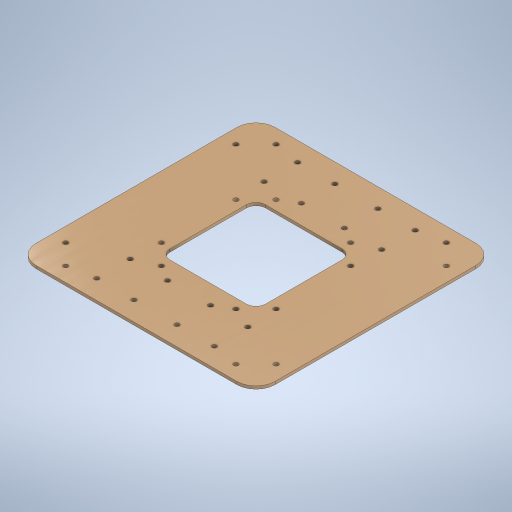
# Autodesk Inventor part: L1 Wood Base Iteration 1
Saved by Autodesk Inventor 2024 (Build 280153000, 153)
## iProperties
Created: 2023-06-26
Part Number: L1 Wood Base Iteration 1
Material: Aluminum 6061
Document SubType Name: Modeling
Designer: AdminForWorker
Density: 2.7 g/cm^3
Appearance: Brindle
Title: base
Author: AdminForWorker
Autodesk Inventor part; units mm, degrees
ref_plane "YZ Plane" through (0, 0, 0) normal (1, 0, 0) x (0, 1, 0)
ref_plane "XZ Plane" through (0, 0, 0) normal (0, 1, 0) x (-1, 0, 0)
ref_plane "XY Plane" through (0, 0, 0) normal (0, 0, 1) x (1, 0, 0)
sketch "Sketch3" plane through (0, 0, 0) normal (0, 1, 0) x (-1, 0, 0)
  line L0 (105, -125) -> (-105, -125)
  line L1 (-125, -105) -> (-125, 105)
  line L2 (-105, 125) -> (105, 125)
  line L3 (125, 105) -> (125, -105)
  line L4 (125, -125) -> (-125, 125) construction
  line L5 (-125, -125) -> (125, 125) construction
  arc A0 (125, 105) -> (105, 125) centre (105, 105) ccw
  arc A1 (105, -125) -> (125, -105) centre (105, -105) ccw
  arc A2 (-105, 125) -> (-125, 105) centre (-105, 105) ccw
  arc A3 (-125, -105) -> (-105, -125) centre (-105, -105) ccw
  line L6 (-40, 50) -> (40, 50)
  line L7 (50, 40) -> (50, -40)
  line L8 (40, -50) -> (-40, -50)
  line L9 (-50, -40) -> (-50, 40)
  line L10 (-50, 50) -> (50, -50) construction
  line L11 (50, 50) -> (-50, -50) construction
  arc A4 (50, 40) -> (40, 50) centre (40, 40) ccw
  arc A5 (-40, 50) -> (-50, 40) centre (-40, 40) ccw
  arc A6 (-50, -40) -> (-40, -50) centre (-40, -40) ccw
  arc A7 (40, -50) -> (50, -40) centre (40, -40) ccw
  point P0 (0, 0)
  dimension "L0" = 250
  dimension "W0" = 250
  dimension "d126" = 20
  dimension "d127" = 100
  dimension "d128" = 100
  dimension "d129" = 10
  constraints: 24 end point, 16 point on circle, 16 point on line, 16 tangent, 8 centre point, 6 equal radius, 4 midpoint, 4 parallel, 2 horizontal, 2 perpendicular
  measures "L0" distance of L4.end L5.end
  measures "W0" distance of L5.start L4.end
  measures "d126" radius of A0
  measures "d127" distance of L10.end L11.end
  measures "d128" distance of L11.start L10.end
  measures "d129" radius of A4
extrude "Main Body Extrusion" add sketch "Sketch3" along normal blind 3
sketch "Sketch11" plane through (0, 3, 0) normal (0, 1, 0) x (1, 0, 0)
  circle A0 centre (61.4917, -70.0531) radius 2.5
  circle A1 centre (22.4917, -105.0531) radius 2.5
  circle A2 centre (-22.5083, -70.0531) radius 2.5
  circle A3 centre (-61.5083, -105.0531) radius 2.5
  circle A4 centre (-22.5083, -105.0531) radius 2.5
  circle A5 centre (61.4917, -105.0531) radius 2.5
  circle A6 centre (-61.5083, -70.0531) radius 2.5
  circle A7 centre (61.4917, 104.9469) radius 2.5
  circle A8 centre (61.4917, 69.9469) radius 2.5
  circle A9 centre (22.4917, 104.9469) radius 2.5
  circle A10 centre (-22.5083, 69.9469) radius 2.5
  circle A11 centre (-61.5083, 104.9469) radius 2.5
  circle A12 centre (-22.5083, 104.9469) radius 2.5
  circle A13 centre (22.4917, -70.0531) radius 2.5
  circle A14 centre (22.4917, 69.9469) radius 2.5
  line L0 (-125.0083, 124.9469) -> (124.9917, 124.9469)
  line L1 (124.9917, 124.9469) -> (124.9917, -125.0531)
  line L2 (124.9917, -125.0531) -> (-125.0083, -125.0531)
  line L3 (-125.0083, -125.0531) -> (-125.0083, 124.9469)
  point P0 (0, 0)
  point P1 (-61.5083, 69.9469)
  dimension "d86" = 250
  dimension "d87" = 250
  constraints: 15 centre point, 15 coincident, 8 end point, 2 parallel, 1 horizontal, 1 horizontal alignment, 1 perpendicular, 1 vertical alignment
  measures "d86" distance of L1.end L2.end
  measures "d87" distance of L0.end L1.end
hole "Bracket Holes" at (61.4917, 3, 70.0531) at (22.4917, 3, 105.0531) at (-22.5083, 3, 70.0531) at (-61.5083, 3, 105.0531) at (-22.5083, 3, 105.0531) at (61.4917, 3, 105.0531) at (-61.5083, 3, 70.0531) at (61.4917, 3, -104.9469) at (61.4917, 3, -69.9469) at (22.4917, 3, -104.9469) at (-22.5083, 3, -69.9469) at (-61.5083, 3, -104.9469) at (-22.5083, 3, -104.9469) at (22.4917, 3, 70.0531) at (22.4917, 3, -69.9469) at (-61.5083, 3, -69.9469) direction (0, -1, 0) diameter 5 end through all
sketch "Sketch12" plane through (0, 3, 0) normal (0, 1, 0) x (1, 0, 0)
  line L0 (85, -115) -> (115, -115)
  line L1 (115, -115) -> (115, -110.5263)
  line L2 (105, -105) -> (85, -105)
  line L3 (85, -105) -> (85, -115)
  line L4 (115, -85) -> (105, -85)
  line L5 (105, -85) -> (105, -105)
  line L6 (110.5263, -115) -> (115, -115)
  line L7 (115, -115) -> (115, -85)
  line L8 (125, -105) -> (125, 105) projected
  line L9 (-105, -125) -> (105, -125) projected
  line L10 (115, 115) -> (110.5263, 115)
  line L11 (115, 110.5263) -> (115, 115)
  line L12 (105, 105) -> (105, 85)
  line L13 (105, 85) -> (115, 85)
  line L14 (115, 85) -> (115, 115)
  line L15 (85, 115) -> (85, 105)
  line L16 (85, 105) -> (105, 105)
  line L17 (115, 115) -> (85, 115)
  line L18 (-115, 115) -> (-115, 110.5263)
  line L19 (-110.5263, 115) -> (-115, 115)
  line L20 (-105, 105) -> (-85, 105)
  line L21 (-85, 105) -> (-85, 115)
  line L22 (-85, 115) -> (-115, 115)
  line L23 (-115, 85) -> (-105, 85)
  line L24 (-105, 85) -> (-105, 105)
  line L25 (-115, 115) -> (-115, 85)
  line L26 (-115, -115) -> (-110.5263, -115)
  line L27 (-115, -110.5263) -> (-115, -115)
  line L28 (-105, -105) -> (-105, -85)
  line L29 (-105, -85) -> (-115, -85)
  line L30 (-115, -85) -> (-115, -115)
  line L31 (-85, -115) -> (-85, -105)
  line L32 (-85, -105) -> (-105, -105)
  line L33 (-115, -115) -> (-85, -115)
  line L34 (35, -65) -> (65, -65)
  line L35 (65, -65) -> (65, -50.5263)
  line L36 (55, -55) -> (35, -55)
  line L37 (35, -55) -> (35, -65)
  line L38 (65, -35) -> (55, -35)
  line L39 (55, -35) -> (55, -55)
  line L40 (66.4138, -65) -> (65, -65)
  line L41 (65, -65) -> (65, -35)
  line L42 (65, 66.4138) -> (65, 65)
  line L43 (65, 65) -> (50.5263, 65)
  line L44 (65, 65) -> (35, 65)
  line L45 (65, 35) -> (65, 65)
  line L46 (35, 55) -> (55, 55)
  line L47 (55, 55) -> (55, 35)
  line L48 (35, 65) -> (35, 55)
  line L49 (55, 35) -> (65, 35)
  line L50 (-66.4138, 65) -> (-65, 65)
  line L51 (-65, 65) -> (-65, 50.5263)
  line L52 (-65, 65) -> (-65, 35)
  line L53 (-35, 65) -> (-65, 65)
  line L54 (-55, 35) -> (-55, 55)
  line L55 (-55, 55) -> (-35, 55)
  line L56 (-65, 35) -> (-55, 35)
  line L57 (-35, 55) -> (-35, 65)
  line L58 (-65, -66.4138) -> (-65, -65)
  line L59 (-65, -65) -> (-50.5263, -65)
  line L60 (-65, -65) -> (-35, -65)
  line L61 (-65, -35) -> (-65, -65)
  line L62 (-35, -55) -> (-55, -55)
  line L63 (-55, -55) -> (-55, -35)
  line L64 (-35, -65) -> (-35, -55)
  line L65 (-55, -35) -> (-65, -35)
  point P0 (0, 0)
  point P1 (125, -125)
  point P2 (125, 125)
  point P3 (-125, -125)
  point P4 (89, -110)
  point P5 (110, -89)
  point P6 (110, -85)
  point P7 (85, 110)
  point P8 (89, 110)
  point P9 (110, 89)
  point P10 (-110, 85)
  point P11 (-110, 89)
  point P12 (-89, 110)
  point P13 (-85, -110)
  point P14 (-89, -110)
  point P15 (-110, -89)
  point P16 (39, -60)
  point P17 (60, -39)
  point P18 (60, -35)
  point P19 (35, 60)
  point P20 (60, 39)
  point P21 (39, 60)
  point P22 (-60, 35)
  point P23 (-39, 60)
  point P24 (-60, 39)
  point P25 (-35, -60)
  point P26 (-60, -39)
  point P27 (-39, -60)
  dimension "d95" = 30
  dimension "d96" = 30
  dimension "d97" = 20
  dimension "d98" = 20
  dimension "d99" = 10
  dimension "d100" = 10
  dimension "d101" = 4
  dimension "d102" = 5
  dimension "d103" = 5
  dimension "d104" = 4
  dimension "d107" = 360
  dimension "d116" = 30
  dimension "d117" = 30
  dimension "d118" = 20
  dimension "d119" = 20
  dimension "d120" = 4
  dimension "d121" = 5
  dimension "d122" = 5
  dimension "d123" = 4
  dimension "d124" = 60
  dimension "d125" = 60
  dimension "d132" = 360
  constraints: 128 end point, 16 point on line, 8 parallel, 4 horizontal, 4 perpendicular, 2 midpoint, 162 other
  measures "d95" distance of L0.start L0.end
  measures "d96" distance of L6.end L4.start
  measures "d97" distance of L2.start L2.end
  measures "d98" distance of L4.end L2.start
  measures "d99" distance between parallel lines of L8 L7
  measures "d100" distance between parallel lines of L9 L0
  measures "d101" distance from line of L3 point (89, -110)
  measures "d102" distance from line of L0 point (89, -110)
  measures "d103" distance from line of L5 point (110, -89)
  measures "d104" distance of point (110, -85) point (110, -89)
  measures "d116" distance of L34.start L34.end
  measures "d117" distance of L40.end L38.start
  measures "d118" distance of L36.start L37.start
  measures "d119" distance of L39.start L36.start
  measures "d120" distance from line of L37 point (39, -60)
  measures "d121" distance from line of L34 point (39, -60)
  measures "d122" distance from line of L39 point (60, -39)
  measures "d123" distance of point (60, -35) point (60, -39)
  measures "d124" distance between parallel lines of L9 L34
  measures "d125" distance between parallel lines of L8 L41
hole "Hole4" at (89, 3, 110) at (110, 3, 89) at (89, 3, -110) at (110, 3, -89) at (-110, 3, -89) at (-89, 3, -110) at (-89, 3, 110) at (-110, 3, 89) at (-60, 3, 39) at (-39, 3, 60) at (-60, 3, -39) at (-39, 3, -60) at (39, 3, -60) at (60, 3, -39) at (60, 3, 39) at (39, 3, 60) direction (0, -1, 0) diameter 5 end through all
